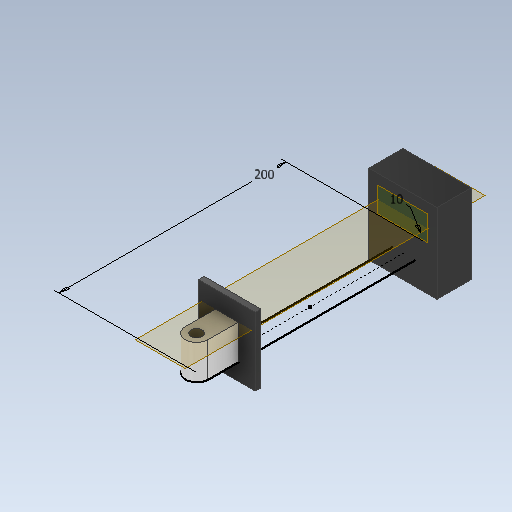
# Autodesk Inventor part: j4 for end effector
Saved by Autodesk Inventor 2020 (Build 240168000, 168)
## iProperties
Created: 2020-07-11
Part Number: j4 for end effector
Material: Aluminum 6061
Document SubType Name: Modeling
Designer: Vikki
Density: 2.7 g/cm^3
Appearance: Glossy - Black
Mass: 430.28 g
Surface Area: 274.098 cm^2
Volume: 159.363 cm^3
Author: Vikki
Autodesk Inventor part; units mm, degrees
ref_plane "YZ Plane" through (0, 0, 0) normal (1, 0, 0) x (0, 1, 0)
ref_plane "XY Plane" through (0, 0, 0) normal (0, 0, 1) x (1, 0, 0)
sketch "Sketch1" plane through (0, 0, 0) normal (0, 1, 0) x (-1, 0, 0)
  line L0 (0, 0) -> (0, -200) construction
  line L1 (-10, 0) -> (-10, -200)
  line L2 (10, -200) -> (10, 0)
  arc A0 (10, 0) -> (-10, 0) centre (0, 0) ccw
  arc A1 (-10, -200) -> (10, -200) centre (0, -200) ccw
  point P0 (0, -100)
  dimension "d0" = 10
  dimension "d1" = 200
  constraints: 8 end point, 4 point on circle, 4 tangent, 2 centre point, 1 midpoint, 1 parallel, 1 vertical
  measures "d0" radius of A1
  measures "d1" distance of L0.start L0.end
ref_plane "Work Plane1" through (0, 30, 0) normal (0, 1, 0) x (-1, 0, 0)
sketch "Sketch2" plane through (0, 30, 0) normal (0, 1, 0) x (-1, 0, 0)
  line L0 (10, -200) -> (10, 0) projected
  arc A0 (10, 0) -> (-10, 0) centre (0, 0) ccw projected
  line L1 (-10, 0) -> (-10, -200) projected
  arc A1 (-10, -200) -> (10, -200) centre (0, -200) ccw projected
  circle A2 centre (0, 0) radius 5
  line L2 (10, -30) -> (-10, -30)
  dimension "d20" = 10
  dimension "d21" = 30
  constraints: 2 end point, 2 point on line, 1 centre point, 1 coincident, 1 perpendicular
  measures "d20" diameter of A2
  measures "d21" distance from line of L2 point (0, 0)
ref_plane "Work Plane2" through (0, 30, -181.6778) normal (0, 0, -1) x (0, -1, 0)
sketch "Sketch4" plane through (0, 30, -181.6778) normal (0, 0, -1) x (0, -1, 0)
  line L0 (33.9, -13.0515) -> (33.9, -6.9485) construction
  line L1 (33.9, -6.9485) -> (36.2985, -4.55) construction
  line L2 (36.2985, -4.55) -> (38.2, -4.55) construction
  line L3 (38.2, -4.55) -> (38.2, -6.9) construction
  line L4 (38.2, -6.9) -> (39.1, -6.9) construction
  line L5 (39.1, -6.9) -> (39.1, -6.6) construction
  arc A0 (39.3, -6.4) -> (39.1, -6.6) centre (39.3, -6.6) ccw construction
  line L6 (39.3, -6.4) -> (40, -6.4) construction
  line L7 (40, -6.4) -> (40, 6.4) construction
  line L8 (40, 6.4) -> (39.3, 6.4) construction
  arc A1 (39.1, 6.6) -> (39.3, 6.4) centre (39.3, 6.6) ccw construction
  line L9 (39.1, 6.6) -> (39.1, 6.9) construction
  line L10 (39.1, 6.9) -> (38.2, 6.9) construction
  line L11 (38.2, 6.9) -> (38.2, 4.55) construction
  line L12 (38.2, 4.55) -> (36.2985, 4.55) construction
  line L13 (36.2985, 4.55) -> (33.9, 6.9485) construction
  line L14 (33.9, 6.9485) -> (33.9, 13.0515) construction
  line L15 (33.9, 13.0515) -> (36.2985, 15.45) construction
  line L16 (36.2985, 15.45) -> (38.2, 15.45) construction
  line L17 (38.2, 15.45) -> (38.2, 13.1) construction
  line L18 (38.2, 13.1) -> (39.1, 13.1) construction
  line L19 (39.1, 13.1) -> (39.1, 13.4) construction
  arc A2 (39.3, 13.6) -> (39.1, 13.4) centre (39.3, 13.4) ccw construction
  line L20 (39.3, 13.6) -> (40, 13.6) construction
  line L21 (40, 13.6) -> (40, 18.5) construction
  arc A3 (40, 18.5) -> (38.5, 20) centre (38.5, 18.5) ccw construction
  line L22 (38.5, 20) -> (33.6, 20) construction
  line L23 (33.6, 20) -> (33.6, 19.3) construction
  arc A4 (33.4, 19.1) -> (33.6, 19.3) centre (33.4, 19.3) ccw construction
  line L24 (33.4, 19.1) -> (33.1, 19.1) construction
  line L25 (33.1, 19.1) -> (33.1, 18.2) construction
  line L26 (33.1, 18.2) -> (35.45, 18.2) construction
  line L27 (35.45, 18.2) -> (35.45, 16.2985) construction
  line L28 (35.45, 16.2985) -> (33.0515, 13.9) construction
  line L29 (33.0515, 13.9) -> (26.9485, 13.9) construction
  line L30 (26.9485, 13.9) -> (24.55, 16.2985) construction
  line L31 (24.55, 16.2985) -> (24.55, 18.2) construction
  line L32 (24.55, 18.2) -> (26.9, 18.2) construction
  line L33 (26.9, 18.2) -> (26.9, 19.1) construction
  line L34 (26.9, 19.1) -> (26.6, 19.1) construction
  arc A5 (26.4, 19.3) -> (26.6, 19.1) centre (26.6, 19.3) ccw construction
  line L35 (26.4, 19.3) -> (26.4, 20) construction
  line L36 (26.4, 20) -> (21.5, 20) construction
  arc A6 (21.5, 20) -> (20, 18.5) centre (21.5, 18.5) ccw construction
  line L37 (20, 18.5) -> (20, 13.6) construction
  line L38 (20, 13.6) -> (20.7, 13.6) construction
  arc A7 (20.9, 13.4) -> (20.7, 13.6) centre (20.7, 13.4) ccw construction
  line L39 (20.9, 13.4) -> (20.9, 13.1) construction
  line L40 (20.9, 13.1) -> (21.8, 13.1) construction
  line L41 (21.8, 13.1) -> (21.8, 15.45) construction
  line L42 (21.8, 15.45) -> (23.7015, 15.45) construction
  line L43 (23.7015, 15.45) -> (26.0515, 13.1) construction
  line L44 (26.0515, 13.1) -> (26.0515, 6.9) construction
  line L45 (26.0515, 6.9) -> (23.7015, 4.55) construction
  line L46 (23.7015, 4.55) -> (21.8, 4.55) construction
  line L47 (21.8, 4.55) -> (21.8, 6.9) construction
  line L48 (21.8, 6.9) -> (20.9, 6.9) construction
  line L49 (20.9, 6.9) -> (20.9, 6.6) construction
  arc A8 (20.7, 6.4) -> (20.9, 6.6) centre (20.7, 6.6) ccw construction
  line L50 (20.7, 6.4) -> (20, 6.4) construction
  line L51 (20, 6.4) -> (20, -6.4) construction
  line L52 (20, -6.4) -> (20.7, -6.4) construction
  arc A9 (20.9, -6.6) -> (20.7, -6.4) centre (20.7, -6.6) ccw construction
  line L53 (20.9, -6.6) -> (20.9, -6.9) construction
  line L54 (20.9, -6.9) -> (21.8, -6.9) construction
  line L55 (21.8, -6.9) -> (21.8, -4.55) construction
  line L56 (21.8, -4.55) -> (23.7015, -4.55) construction
  line L57 (23.7015, -4.55) -> (26.0515, -6.9) construction
  line L58 (26.0515, -6.9) -> (26.0515, -13.1) construction
  line L59 (26.0515, -13.1) -> (23.7015, -15.45) construction
  line L60 (23.7015, -15.45) -> (21.8, -15.45) construction
  line L61 (21.8, -15.45) -> (21.8, -13.1) construction
  line L62 (21.8, -13.1) -> (20.9, -13.1) construction
  line L63 (20.9, -13.1) -> (20.9, -13.4) construction
  arc A10 (20.7, -13.6) -> (20.9, -13.4) centre (20.7, -13.4) ccw construction
  line L64 (20.7, -13.6) -> (20, -13.6) construction
  line L65 (20, -13.6) -> (20, -18.5) construction
  arc A11 (20, -18.5) -> (21.5, -20) centre (21.5, -18.5) ccw construction
  line L66 (21.5, -20) -> (26.4, -20) construction
  line L67 (26.4, -20) -> (26.4, -19.3) construction
  arc A12 (26.6, -19.1) -> (26.4, -19.3) centre (26.6, -19.3) ccw construction
  line L68 (26.6, -19.1) -> (26.9, -19.1) construction
  line L69 (26.9, -19.1) -> (26.9, -18.2) construction
  line L70 (26.9, -18.2) -> (24.55, -18.2) construction
  line L71 (24.55, -18.2) -> (24.55, -16.2985) construction
  line L72 (24.55, -16.2985) -> (26.9485, -13.9) construction
  line L73 (26.9485, -13.9) -> (33.0515, -13.9) construction
  line L74 (33.0515, -13.9) -> (35.45, -16.2985) construction
  line L75 (35.45, -16.2985) -> (35.45, -18.2) construction
  line L76 (35.45, -18.2) -> (33.1, -18.2) construction
  line L77 (33.1, -18.2) -> (33.1, -19.1) construction
  line L78 (33.1, -19.1) -> (33.4, -19.1) construction
  arc A13 (33.6, -19.3) -> (33.4, -19.1) centre (33.4, -19.3) ccw construction
  line L79 (33.6, -19.3) -> (33.6, -20) construction
  line L80 (33.6, -20) -> (38.5, -20) construction
  arc A14 (38.5, -20) -> (40, -18.5) centre (38.5, -18.5) ccw construction
  line L81 (40, -18.5) -> (40, -13.6) construction
  line L82 (40, -13.6) -> (39.3, -13.6) construction
  arc A15 (39.1, -13.4) -> (39.3, -13.6) centre (39.3, -13.4) ccw construction
  line L83 (39.1, -13.4) -> (39.1, -13.1) construction
  line L84 (39.1, -13.1) -> (38.2, -13.1) construction
  line L85 (38.2, -13.1) -> (38.2, -15.45) construction
  line L86 (38.2, -15.45) -> (36.2985, -15.45) construction
  line L87 (36.2985, -15.45) -> (33.9, -13.0515) construction
  circle A16 centre (30, 10) radius 2.5 construction
  circle A17 centre (30, -10) radius 2.5 construction
  line L88 (33.0515, 6.1) -> (35.8015, 3.35) construction
  line L89 (35.8015, 3.35) -> (38.2, 3.35) construction
  line L90 (38.2, 3.35) -> (38.2, -3.35) construction
  line L91 (38.2, -3.35) -> (35.8015, -3.35) construction
  line L92 (35.8015, -3.35) -> (33.0515, -6.1) construction
  line L93 (33.0515, -6.1) -> (26.9485, -6.1) construction
  line L94 (26.9485, -6.1) -> (24.1985, -3.35) construction
  line L95 (24.1985, -3.35) -> (21.8, -3.35) construction
  line L96 (21.8, -3.35) -> (21.8, 3.35) construction
  line L97 (21.8, 3.35) -> (24.1985, 3.35) construction
  line L98 (24.1985, 3.35) -> (26.9485, 6.1) construction
  line L99 (26.9485, 6.1) -> (33.0515, 6.1) construction
  line L100 (3.9, -13.0515) -> (3.9, -6.9485) construction
  line L101 (3.9, -6.9485) -> (6.2985, -4.55) construction
  line L102 (6.2985, -4.55) -> (8.2, -4.55) construction
  line L103 (8.2, -4.55) -> (8.2, -6.9) construction
  line L104 (8.2, -6.9) -> (9.1, -6.9) construction
  line L105 (9.1, -6.9) -> (9.1, -6.6) construction
  arc A18 (9.3, -6.4) -> (9.1, -6.6) centre (9.3, -6.6) ccw construction
  line L106 (9.3, -6.4) -> (10, -6.4) construction
  line L107 (10, -6.4) -> (10, 6.4) construction
  line L108 (10, 6.4) -> (9.3, 6.4) construction
  arc A19 (9.1, 6.6) -> (9.3, 6.4) centre (9.3, 6.6) ccw construction
  line L109 (9.1, 6.6) -> (9.1, 6.9) construction
  line L110 (9.1, 6.9) -> (8.2, 6.9) construction
  line L111 (8.2, 6.9) -> (8.2, 4.55) construction
  line L112 (8.2, 4.55) -> (6.2985, 4.55) construction
  line L113 (6.2985, 4.55) -> (3.9, 6.9485) construction
  line L114 (3.9, 6.9485) -> (3.9, 13.0515) construction
  line L115 (3.9, 13.0515) -> (6.2985, 15.45) construction
  line L116 (6.2985, 15.45) -> (8.2, 15.45) construction
  line L117 (8.2, 15.45) -> (8.2, 13.1) construction
  line L118 (8.2, 13.1) -> (9.1, 13.1) construction
  line L119 (9.1, 13.1) -> (9.1, 13.4) construction
  arc A20 (9.3, 13.6) -> (9.1, 13.4) centre (9.3, 13.4) ccw construction
  line L120 (9.3, 13.6) -> (10, 13.6) construction
  line L121 (10, 13.6) -> (10, 18.5) construction
  arc A21 (10, 18.5) -> (8.5, 20) centre (8.5, 18.5) ccw construction
  line L122 (8.5, 20) -> (3.6, 20) construction
  line L123 (3.6, 20) -> (3.6, 19.3) construction
  arc A22 (3.4, 19.1) -> (3.6, 19.3) centre (3.4, 19.3) ccw construction
  line L124 (3.4, 19.1) -> (3.1, 19.1) construction
  line L125 (3.1, 19.1) -> (3.1, 18.2) construction
  line L126 (3.1, 18.2) -> (5.45, 18.2) construction
  line L127 (5.45, 18.2) -> (5.45, 16.2985) construction
  line L128 (5.45, 16.2985) -> (3.0515, 13.9) construction
  line L129 (3.0515, 13.9) -> (-3.0515, 13.9) construction
  line L130 (-3.0515, 13.9) -> (-5.45, 16.2985) construction
  line L131 (-5.45, 16.2985) -> (-5.45, 18.2) construction
  line L132 (-5.45, 18.2) -> (-3.1, 18.2) construction
  line L133 (-3.1, 18.2) -> (-3.1, 19.1) construction
  line L134 (-3.1, 19.1) -> (-3.4, 19.1) construction
  arc A23 (-3.6, 19.3) -> (-3.4, 19.1) centre (-3.4, 19.3) ccw construction
  line L135 (-3.6, 19.3) -> (-3.6, 20) construction
  line L136 (-3.6, 20) -> (-8.5, 20) construction
  arc A24 (-8.5, 20) -> (-10, 18.5) centre (-8.5, 18.5) ccw construction
  line L137 (-10, 18.5) -> (-10, 13.6) construction
  line L138 (-10, 13.6) -> (-9.3, 13.6) construction
  arc A25 (-9.1, 13.4) -> (-9.3, 13.6) centre (-9.3, 13.4) ccw construction
  line L139 (-9.1, 13.4) -> (-9.1, 13.1) construction
  line L140 (-9.1, 13.1) -> (-8.2, 13.1) construction
  line L141 (-8.2, 13.1) -> (-8.2, 15.45) construction
  line L142 (-8.2, 15.45) -> (-6.2985, 15.45) construction
  line L143 (-6.2985, 15.45) -> (-3.9485, 13.1) construction
  line L144 (-3.9485, 13.1) -> (-3.9485, 6.9) construction
  line L145 (-3.9485, 6.9) -> (-6.2985, 4.55) construction
  line L146 (-6.2985, 4.55) -> (-8.2, 4.55) construction
  line L147 (-8.2, 4.55) -> (-8.2, 6.9) construction
  line L148 (-8.2, 6.9) -> (-9.1, 6.9) construction
  line L149 (-9.1, 6.9) -> (-9.1, 6.6) construction
  arc A26 (-9.3, 6.4) -> (-9.1, 6.6) centre (-9.3, 6.6) ccw construction
  line L150 (-9.3, 6.4) -> (-10, 6.4) construction
  line L151 (-10, 6.4) -> (-10, -6.4) construction
  line L152 (-10, -6.4) -> (-9.3, -6.4) construction
  arc A27 (-9.1, -6.6) -> (-9.3, -6.4) centre (-9.3, -6.6) ccw construction
  line L153 (-9.1, -6.6) -> (-9.1, -6.9) construction
  line L154 (-9.1, -6.9) -> (-8.2, -6.9) construction
  line L155 (-8.2, -6.9) -> (-8.2, -4.55) construction
  line L156 (-8.2, -4.55) -> (-6.2985, -4.55) construction
  line L157 (-6.2985, -4.55) -> (-3.9485, -6.9) construction
  line L158 (-3.9485, -6.9) -> (-3.9485, -13.1) construction
  line L159 (-3.9485, -13.1) -> (-6.2985, -15.45) construction
  line L160 (-6.2985, -15.45) -> (-8.2, -15.45) construction
  line L161 (-8.2, -15.45) -> (-8.2, -13.1) construction
  line L162 (-8.2, -13.1) -> (-9.1, -13.1) construction
  line L163 (-9.1, -13.1) -> (-9.1, -13.4) construction
  arc A28 (-9.3, -13.6) -> (-9.1, -13.4) centre (-9.3, -13.4) ccw construction
  line L164 (-9.3, -13.6) -> (-10, -13.6) construction
  line L165 (-10, -13.6) -> (-10, -18.5) construction
  arc A29 (-10, -18.5) -> (-8.5, -20) centre (-8.5, -18.5) ccw construction
  line L166 (-8.5, -20) -> (-3.6, -20) construction
  line L167 (-3.6, -20) -> (-3.6, -19.3) construction
  arc A30 (-3.4, -19.1) -> (-3.6, -19.3) centre (-3.4, -19.3) ccw construction
  line L168 (-3.4, -19.1) -> (-3.1, -19.1) construction
  line L169 (-3.1, -19.1) -> (-3.1, -18.2) construction
  line L170 (-3.1, -18.2) -> (-5.45, -18.2) construction
  line L171 (-5.45, -18.2) -> (-5.45, -16.2985) construction
  line L172 (-5.45, -16.2985) -> (-3.0515, -13.9) construction
  line L173 (-3.0515, -13.9) -> (3.0515, -13.9) construction
  line L174 (3.0515, -13.9) -> (5.45, -16.2985) construction
  line L175 (5.45, -16.2985) -> (5.45, -18.2) construction
  line L176 (5.45, -18.2) -> (3.1, -18.2) construction
  line L177 (3.1, -18.2) -> (3.1, -19.1) construction
  line L178 (3.1, -19.1) -> (3.4, -19.1) construction
  arc A31 (3.6, -19.3) -> (3.4, -19.1) centre (3.4, -19.3) ccw construction
  line L179 (3.6, -19.3) -> (3.6, -20) construction
  line L180 (3.6, -20) -> (8.5, -20) construction
  arc A32 (8.5, -20) -> (10, -18.5) centre (8.5, -18.5) ccw construction
  line L181 (10, -18.5) -> (10, -13.6) construction
  line L182 (10, -13.6) -> (9.3, -13.6) construction
  arc A33 (9.1, -13.4) -> (9.3, -13.6) centre (9.3, -13.4) ccw construction
  line L183 (9.1, -13.4) -> (9.1, -13.1) construction
  line L184 (9.1, -13.1) -> (8.2, -13.1) construction
  line L185 (8.2, -13.1) -> (8.2, -15.45) construction
  line L186 (8.2, -15.45) -> (6.2985, -15.45) construction
  line L187 (6.2985, -15.45) -> (3.9, -13.0515) construction
  circle A34 centre (0, 10) radius 2.5 construction
  circle A35 centre (0, -10) radius 2.5 construction
  line L188 (3.0515, 6.1) -> (5.8015, 3.35) construction
  line L189 (5.8015, 3.35) -> (8.2, 3.35) construction
  line L190 (8.2, 3.35) -> (8.2, -3.35) construction
  line L191 (8.2, -3.35) -> (5.8015, -3.35) construction
  line L192 (5.8015, -3.35) -> (3.0515, -6.1) construction
  line L193 (3.0515, -6.1) -> (-3.0515, -6.1) construction
  line L194 (-3.0515, -6.1) -> (-5.8015, -3.35) construction
  line L195 (-5.8015, -3.35) -> (-8.2, -3.35) construction
  line L196 (-8.2, -3.35) -> (-8.2, 3.35) construction
  line L197 (-8.2, 3.35) -> (-5.8015, 3.35) construction
  line L198 (-5.8015, 3.35) -> (-3.0515, 6.1) construction
  line L199 (-3.0515, 6.1) -> (3.0515, 6.1) construction
  line L200 (-3.6, 20) -> (33.6, 20) construction
  line L201 (40, 13.6) -> (40, -13.6) construction
  line L202 (33.6, -20) -> (-3.6, -20) construction
  line L203 (-10, -13.6) -> (-10, 13.6) construction
  line L204 (-20, 30) -> (50, 30)
  line L205 (50, 30) -> (50, -30)
  line L206 (50, -30) -> (-20, -30)
  line L207 (-20, -30) -> (-20, 30)
  point P0 (30, 0)
  dimension "d7" = 10
  dimension "d8" = 10
  dimension "d9" = 10
  dimension "d10" = 10
  constraints: 16 end point, 3 perpendicular, 2 collinear, 2 parallel, 1 horizontal
  measures "d7" distance between parallel lines of L205 L201
  measures "d8" distance between parallel lines of L204 L200
  measures "d9" distance between parallel lines of L206 L202
  measures "d10" distance between parallel lines of L207 L203
extrude "Extrusion2" add sketch "Sketch4" along normal blind 30
ref_plane "Work Plane3" through (0, 0, -31.6778) normal (0, 0, 1) x (0, 1, 0)
sketch "Sketch5" plane through (0, 0, -31.6778) normal (0, 0, 1) x (0, 1, 0)
  line L0 (-15, 25) -> (45, 25)
  line L1 (45, 25) -> (45, -25)
  line L2 (45, -25) -> (-15, -25)
  line L3 (-15, -25) -> (-15, 25)
  line L4 (26.1, -6.9485) -> (26.1, -13.0515) construction
  line L5 (26.1, -13.0515) -> (23.7015, -15.45) construction
  line L6 (23.7015, -15.45) -> (21.8, -15.45) construction
  line L7 (21.8, -15.45) -> (21.8, -13.1) construction
  line L8 (21.8, -13.1) -> (20.9, -13.1) construction
  line L9 (20.9, -13.1) -> (20.9, -13.4) construction
  arc A0 (20.7, -13.6) -> (20.9, -13.4) centre (20.7, -13.4) ccw construction
  line L10 (20.7, -13.6) -> (20, -13.6) construction
  line L11 (20, -13.6) -> (20, -18.5) construction
  arc A1 (20, -18.5) -> (21.5, -20) centre (21.5, -18.5) ccw construction
  line L12 (21.5, -20) -> (26.4, -20) construction
  line L13 (26.4, -20) -> (26.4, -19.3) construction
  arc A2 (26.6, -19.1) -> (26.4, -19.3) centre (26.6, -19.3) ccw construction
  line L14 (26.6, -19.1) -> (26.9, -19.1) construction
  line L15 (26.9, -19.1) -> (26.9, -18.2) construction
  line L16 (26.9, -18.2) -> (24.55, -18.2) construction
  line L17 (24.55, -18.2) -> (24.55, -16.2985) construction
  line L18 (24.55, -16.2985) -> (26.9485, -13.9) construction
  line L19 (26.9485, -13.9) -> (33.0515, -13.9) construction
  line L20 (33.0515, -13.9) -> (35.45, -16.2985) construction
  line L21 (35.45, -16.2985) -> (35.45, -18.2) construction
  line L22 (35.45, -18.2) -> (33.1, -18.2) construction
  line L23 (33.1, -18.2) -> (33.1, -19.1) construction
  line L24 (33.1, -19.1) -> (33.4, -19.1) construction
  arc A3 (33.6, -19.3) -> (33.4, -19.1) centre (33.4, -19.3) ccw construction
  line L25 (33.6, -19.3) -> (33.6, -20) construction
  line L26 (33.6, -20) -> (38.5, -20) construction
  arc A4 (38.5, -20) -> (40, -18.5) centre (38.5, -18.5) ccw construction
  line L27 (40, -18.5) -> (40, -13.6) construction
  line L28 (40, -13.6) -> (39.3, -13.6) construction
  arc A5 (39.1, -13.4) -> (39.3, -13.6) centre (39.3, -13.4) ccw construction
  line L29 (39.1, -13.4) -> (39.1, -13.1) construction
  line L30 (39.1, -13.1) -> (38.2, -13.1) construction
  line L31 (38.2, -13.1) -> (38.2, -15.45) construction
  line L32 (38.2, -15.45) -> (36.2985, -15.45) construction
  line L33 (36.2985, -15.45) -> (33.9485, -13.1) construction
  line L34 (33.9485, -13.1) -> (33.9485, -6.9) construction
  line L35 (33.9485, -6.9) -> (36.2985, -4.55) construction
  line L36 (36.2985, -4.55) -> (38.2, -4.55) construction
  line L37 (38.2, -4.55) -> (38.2, -6.9) construction
  line L38 (38.2, -6.9) -> (39.1, -6.9) construction
  line L39 (39.1, -6.9) -> (39.1, -6.6) construction
  arc A6 (39.3, -6.4) -> (39.1, -6.6) centre (39.3, -6.6) ccw construction
  line L40 (39.3, -6.4) -> (40, -6.4) construction
  line L41 (40, -6.4) -> (40, 6.4) construction
  line L42 (40, 6.4) -> (39.3, 6.4) construction
  arc A7 (39.1, 6.6) -> (39.3, 6.4) centre (39.3, 6.6) ccw construction
  line L43 (39.1, 6.6) -> (39.1, 6.9) construction
  line L44 (39.1, 6.9) -> (38.2, 6.9) construction
  line L45 (38.2, 6.9) -> (38.2, 4.55) construction
  line L46 (38.2, 4.55) -> (36.2985, 4.55) construction
  line L47 (36.2985, 4.55) -> (33.9485, 6.9) construction
  line L48 (33.9485, 6.9) -> (33.9485, 13.1) construction
  line L49 (33.9485, 13.1) -> (36.2985, 15.45) construction
  line L50 (36.2985, 15.45) -> (38.2, 15.45) construction
  line L51 (38.2, 15.45) -> (38.2, 13.1) construction
  line L52 (38.2, 13.1) -> (39.1, 13.1) construction
  line L53 (39.1, 13.1) -> (39.1, 13.4) construction
  arc A8 (39.3, 13.6) -> (39.1, 13.4) centre (39.3, 13.4) ccw construction
  line L54 (39.3, 13.6) -> (40, 13.6) construction
  line L55 (40, 13.6) -> (40, 18.5) construction
  arc A9 (40, 18.5) -> (38.5, 20) centre (38.5, 18.5) ccw construction
  line L56 (38.5, 20) -> (33.6, 20) construction
  line L57 (33.6, 20) -> (33.6, 19.3) construction
  arc A10 (33.4, 19.1) -> (33.6, 19.3) centre (33.4, 19.3) ccw construction
  line L58 (33.4, 19.1) -> (33.1, 19.1) construction
  line L59 (33.1, 19.1) -> (33.1, 18.2) construction
  line L60 (33.1, 18.2) -> (35.45, 18.2) construction
  line L61 (35.45, 18.2) -> (35.45, 16.2985) construction
  line L62 (35.45, 16.2985) -> (33.0515, 13.9) construction
  line L63 (33.0515, 13.9) -> (26.9485, 13.9) construction
  line L64 (26.9485, 13.9) -> (24.55, 16.2985) construction
  line L65 (24.55, 16.2985) -> (24.55, 18.2) construction
  line L66 (24.55, 18.2) -> (26.9, 18.2) construction
  line L67 (26.9, 18.2) -> (26.9, 19.1) construction
  line L68 (26.9, 19.1) -> (26.6, 19.1) construction
  arc A11 (26.4, 19.3) -> (26.6, 19.1) centre (26.6, 19.3) ccw construction
  line L69 (26.4, 19.3) -> (26.4, 20) construction
  line L70 (26.4, 20) -> (21.5, 20) construction
  arc A12 (21.5, 20) -> (20, 18.5) centre (21.5, 18.5) ccw construction
  line L71 (20, 18.5) -> (20, 13.6) construction
  line L72 (20, 13.6) -> (20.7, 13.6) construction
  arc A13 (20.9, 13.4) -> (20.7, 13.6) centre (20.7, 13.4) ccw construction
  line L73 (20.9, 13.4) -> (20.9, 13.1) construction
  line L74 (20.9, 13.1) -> (21.8, 13.1) construction
  line L75 (21.8, 13.1) -> (21.8, 15.45) construction
  line L76 (21.8, 15.45) -> (23.7015, 15.45) construction
  line L77 (23.7015, 15.45) -> (26.1, 13.0515) construction
  line L78 (26.1, 13.0515) -> (26.1, 6.9485) construction
  line L79 (26.1, 6.9485) -> (23.7015, 4.55) construction
  line L80 (23.7015, 4.55) -> (21.8, 4.55) construction
  line L81 (21.8, 4.55) -> (21.8, 6.9) construction
  line L82 (21.8, 6.9) -> (20.9, 6.9) construction
  line L83 (20.9, 6.9) -> (20.9, 6.6) construction
  arc A14 (20.7, 6.4) -> (20.9, 6.6) centre (20.7, 6.6) ccw construction
  line L84 (20.7, 6.4) -> (20, 6.4) construction
  line L85 (20, 6.4) -> (20, -6.4) construction
  line L86 (20, -6.4) -> (20.7, -6.4) construction
  arc A15 (20.9, -6.6) -> (20.7, -6.4) centre (20.7, -6.6) ccw construction
  line L87 (20.9, -6.6) -> (20.9, -6.9) construction
  line L88 (20.9, -6.9) -> (21.8, -6.9) construction
  line L89 (21.8, -6.9) -> (21.8, -4.55) construction
  line L90 (21.8, -4.55) -> (23.7015, -4.55) construction
  line L91 (23.7015, -4.55) -> (26.1, -6.9485) construction
  circle A16 centre (30, 10) radius 2.5 construction
  circle A17 centre (30, -10) radius 2.5 construction
  line L92 (24.1985, 3.35) -> (26.9485, 6.1) construction
  line L93 (26.9485, 6.1) -> (33.0515, 6.1) construction
  line L94 (33.0515, 6.1) -> (35.8015, 3.35) construction
  line L95 (35.8015, 3.35) -> (38.2, 3.35) construction
  line L96 (38.2, 3.35) -> (38.2, -3.35) construction
  line L97 (38.2, -3.35) -> (35.8015, -3.35) construction
  line L98 (35.8015, -3.35) -> (33.0515, -6.1) construction
  line L99 (33.0515, -6.1) -> (26.9485, -6.1) construction
  line L100 (26.9485, -6.1) -> (24.1985, -3.35) construction
  line L101 (24.1985, -3.35) -> (21.8, -3.35) construction
  line L102 (21.8, -3.35) -> (21.8, 3.35) construction
  line L103 (21.8, 3.35) -> (24.1985, 3.35) construction
  line L104 (-3.9, -6.9485) -> (-3.9, -13.0515) construction
  line L105 (-3.9, -13.0515) -> (-6.2985, -15.45) construction
  line L106 (-6.2985, -15.45) -> (-8.2, -15.45) construction
  line L107 (-8.2, -15.45) -> (-8.2, -13.1) construction
  line L108 (-8.2, -13.1) -> (-9.1, -13.1) construction
  line L109 (-9.1, -13.1) -> (-9.1, -13.4) construction
  arc A18 (-9.3, -13.6) -> (-9.1, -13.4) centre (-9.3, -13.4) ccw construction
  line L110 (-9.3, -13.6) -> (-10, -13.6) construction
  line L111 (-10, -13.6) -> (-10, -18.5) construction
  arc A19 (-10, -18.5) -> (-8.5, -20) centre (-8.5, -18.5) ccw construction
  line L112 (-8.5, -20) -> (-3.6, -20) construction
  line L113 (-3.6, -20) -> (-3.6, -19.3) construction
  arc A20 (-3.4, -19.1) -> (-3.6, -19.3) centre (-3.4, -19.3) ccw construction
  line L114 (-3.4, -19.1) -> (-3.1, -19.1) construction
  line L115 (-3.1, -19.1) -> (-3.1, -18.2) construction
  line L116 (-3.1, -18.2) -> (-5.45, -18.2) construction
  line L117 (-5.45, -18.2) -> (-5.45, -16.2985) construction
  line L118 (-5.45, -16.2985) -> (-3.0515, -13.9) construction
  line L119 (-3.0515, -13.9) -> (3.0515, -13.9) construction
  line L120 (3.0515, -13.9) -> (5.45, -16.2985) construction
  line L121 (5.45, -16.2985) -> (5.45, -18.2) construction
  line L122 (5.45, -18.2) -> (3.1, -18.2) construction
  line L123 (3.1, -18.2) -> (3.1, -19.1) construction
  line L124 (3.1, -19.1) -> (3.4, -19.1) construction
  arc A21 (3.6, -19.3) -> (3.4, -19.1) centre (3.4, -19.3) ccw construction
  line L125 (3.6, -19.3) -> (3.6, -20) construction
  line L126 (3.6, -20) -> (8.5, -20) construction
  arc A22 (8.5, -20) -> (10, -18.5) centre (8.5, -18.5) ccw construction
  line L127 (10, -18.5) -> (10, -13.6) construction
  line L128 (10, -13.6) -> (9.3, -13.6) construction
  arc A23 (9.1, -13.4) -> (9.3, -13.6) centre (9.3, -13.4) ccw construction
  line L129 (9.1, -13.4) -> (9.1, -13.1) construction
  line L130 (9.1, -13.1) -> (8.2, -13.1) construction
  line L131 (8.2, -13.1) -> (8.2, -15.45) construction
  line L132 (8.2, -15.45) -> (6.2985, -15.45) construction
  line L133 (6.2985, -15.45) -> (3.9485, -13.1) construction
  line L134 (3.9485, -13.1) -> (3.9485, -6.9) construction
  line L135 (3.9485, -6.9) -> (6.2985, -4.55) construction
  line L136 (6.2985, -4.55) -> (8.2, -4.55) construction
  line L137 (8.2, -4.55) -> (8.2, -6.9) construction
  line L138 (8.2, -6.9) -> (9.1, -6.9) construction
  line L139 (9.1, -6.9) -> (9.1, -6.6) construction
  arc A24 (9.3, -6.4) -> (9.1, -6.6) centre (9.3, -6.6) ccw construction
  line L140 (9.3, -6.4) -> (10, -6.4) construction
  line L141 (10, -6.4) -> (10, 6.4) construction
  line L142 (10, 6.4) -> (9.3, 6.4) construction
  arc A25 (9.1, 6.6) -> (9.3, 6.4) centre (9.3, 6.6) ccw construction
  line L143 (9.1, 6.6) -> (9.1, 6.9) construction
  line L144 (9.1, 6.9) -> (8.2, 6.9) construction
  line L145 (8.2, 6.9) -> (8.2, 4.55) construction
  line L146 (8.2, 4.55) -> (6.2985, 4.55) construction
  line L147 (6.2985, 4.55) -> (3.9485, 6.9) construction
  line L148 (3.9485, 6.9) -> (3.9485, 13.1) construction
  line L149 (3.9485, 13.1) -> (6.2985, 15.45) construction
  line L150 (6.2985, 15.45) -> (8.2, 15.45) construction
  line L151 (8.2, 15.45) -> (8.2, 13.1) construction
  line L152 (8.2, 13.1) -> (9.1, 13.1) construction
  line L153 (9.1, 13.1) -> (9.1, 13.4) construction
  arc A26 (9.3, 13.6) -> (9.1, 13.4) centre (9.3, 13.4) ccw construction
  line L154 (9.3, 13.6) -> (10, 13.6) construction
  line L155 (10, 13.6) -> (10, 18.5) construction
  arc A27 (10, 18.5) -> (8.5, 20) centre (8.5, 18.5) ccw construction
  line L156 (8.5, 20) -> (3.6, 20) construction
  line L157 (3.6, 20) -> (3.6, 19.3) construction
  arc A28 (3.4, 19.1) -> (3.6, 19.3) centre (3.4, 19.3) ccw construction
  line L158 (3.4, 19.1) -> (3.1, 19.1) construction
  line L159 (3.1, 19.1) -> (3.1, 18.2) construction
  line L160 (3.1, 18.2) -> (5.45, 18.2) construction
  line L161 (5.45, 18.2) -> (5.45, 16.2985) construction
  line L162 (5.45, 16.2985) -> (3.0515, 13.9) construction
  line L163 (3.0515, 13.9) -> (-3.0515, 13.9) construction
  line L164 (-3.0515, 13.9) -> (-5.45, 16.2985) construction
  line L165 (-5.45, 16.2985) -> (-5.45, 18.2) construction
  line L166 (-5.45, 18.2) -> (-3.1, 18.2) construction
  line L167 (-3.1, 18.2) -> (-3.1, 19.1) construction
  line L168 (-3.1, 19.1) -> (-3.4, 19.1) construction
  arc A29 (-3.6, 19.3) -> (-3.4, 19.1) centre (-3.4, 19.3) ccw construction
  line L169 (-3.6, 19.3) -> (-3.6, 20) construction
  line L170 (-3.6, 20) -> (-8.5, 20) construction
  arc A30 (-8.5, 20) -> (-10, 18.5) centre (-8.5, 18.5) ccw construction
  line L171 (-10, 18.5) -> (-10, 13.6) construction
  line L172 (-10, 13.6) -> (-9.3, 13.6) construction
  arc A31 (-9.1, 13.4) -> (-9.3, 13.6) centre (-9.3, 13.4) ccw construction
  line L173 (-9.1, 13.4) -> (-9.1, 13.1) construction
  line L174 (-9.1, 13.1) -> (-8.2, 13.1) construction
  line L175 (-8.2, 13.1) -> (-8.2, 15.45) construction
  line L176 (-8.2, 15.45) -> (-6.2985, 15.45) construction
  line L177 (-6.2985, 15.45) -> (-3.9, 13.0515) construction
  line L178 (-3.9, 13.0515) -> (-3.9, 6.9485) construction
  line L179 (-3.9, 6.9485) -> (-6.2985, 4.55) construction
  line L180 (-6.2985, 4.55) -> (-8.2, 4.55) construction
  line L181 (-8.2, 4.55) -> (-8.2, 6.9) construction
  line L182 (-8.2, 6.9) -> (-9.1, 6.9) construction
  line L183 (-9.1, 6.9) -> (-9.1, 6.6) construction
  arc A32 (-9.3, 6.4) -> (-9.1, 6.6) centre (-9.3, 6.6) ccw construction
  line L184 (-9.3, 6.4) -> (-10, 6.4) construction
  line L185 (-10, 6.4) -> (-10, -6.4) construction
  line L186 (-10, -6.4) -> (-9.3, -6.4) construction
  arc A33 (-9.1, -6.6) -> (-9.3, -6.4) centre (-9.3, -6.6) ccw construction
  line L187 (-9.1, -6.6) -> (-9.1, -6.9) construction
  line L188 (-9.1, -6.9) -> (-8.2, -6.9) construction
  line L189 (-8.2, -6.9) -> (-8.2, -4.55) construction
  line L190 (-8.2, -4.55) -> (-6.2985, -4.55) construction
  line L191 (-6.2985, -4.55) -> (-3.9, -6.9485) construction
  circle A34 centre (0, 10) radius 2.5 construction
  circle A35 centre (0, -10) radius 2.5 construction
  line L192 (-5.8015, 3.35) -> (-3.0515, 6.1) construction
  line L193 (-3.0515, 6.1) -> (3.0515, 6.1) construction
  line L194 (3.0515, 6.1) -> (5.8015, 3.35) construction
  line L195 (5.8015, 3.35) -> (8.2, 3.35) construction
  line L196 (8.2, 3.35) -> (8.2, -3.35) construction
  line L197 (8.2, -3.35) -> (5.8015, -3.35) construction
  line L198 (5.8015, -3.35) -> (3.0515, -6.1) construction
  line L199 (3.0515, -6.1) -> (-3.0515, -6.1) construction
  line L200 (-3.0515, -6.1) -> (-5.8015, -3.35) construction
  line L201 (-5.8015, -3.35) -> (-8.2, -3.35) construction
  line L202 (-8.2, -3.35) -> (-8.2, 3.35) construction
  line L203 (-8.2, 3.35) -> (-5.8015, 3.35) construction
  point P0 (0, 0)
  dimension "d13" = 5
  dimension "d15" = 5
  dimension "d16" = 5
  dimension "d17" = 5
  constraints: 8 end point, 2 parallel, 1 horizontal, 1 perpendicular
  measures "d13" distance between parallel lines of L26 L2
  measures "d15" distance between parallel lines of L0 L56
  measures "d16" distance between parallel lines of L1 L41
  measures "d17" distance between parallel lines of L3 L185
extrude "Extrusion3" add sketch "Sketch5" along normal blind 5
extrude "Extrusion4" add sketch "Sketch2" against normal blind 30 contours L2 L1 A0 L0
body "Solid1"
